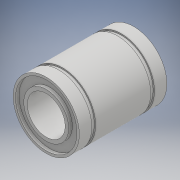
# Autodesk Inventor part: rolamento_linear_lm16uu.iam
Saved by Autodesk Inventor 2018 (Build 220112000, 112)
## iProperties
Created: 2018-05-16
Part Number: rolamento_linear_lm16uu.iam
Material: Genérico
Document SubType Name: Modeling
Designer: Usuario
Density: 1 g/cm^3
Appearance: Padrão
Mass: 6.471 g
Surface Area: 72.2059 cm^2
Volume: 6.471 cm^3
Author: Usuario
Autodesk Inventor part; units mm, degrees
ref_plane "YZ Plane" through (0, 0, 0) normal (1, 0, 0) x (0, 1, 0)
ref_plane "XZ Plane" through (0, 0, 0) normal (0, 1, 0) x (-1, 0, 0)
ref_plane "XY Plane" through (0, 0, 0) normal (0, 0, 1) x (1, 0, 0)
sketch "Esboço1" plane through (0, 0, 0) normal (0, 0, 1) x (1, 0, 0)
  line L0 (-14, 0) -> (-14, 5.25)
  line L1 (-14, 5.25) -> (-13.45, 5.25)
  line L2 (-13.45, 5.25) -> (-13.45, 6.85)
  line L3 (-13.45, 6.85) -> (-14, 6.85)
  line L4 (-14, 6.85) -> (-14, 30.15)
  line L5 (-14, 30.15) -> (-13.45, 30.15)
  line L6 (-13.45, 30.15) -> (-13.45, 31.75)
  line L7 (-13.45, 31.75) -> (-14, 31.75)
  line L8 (-14, 31.75) -> (-14, 37)
  line L9 (-14, 37) -> (-13, 37)
  line L10 (-14, 0) -> (-13, 0)
  line L11 (-13, 0) -> (0, 0) construction
  line L12 (0, 0) -> (0, 37) construction
  line L13 (0, 37) -> (-13, 37) construction
  line L14 (-13, 37) -> (-13, 0)
  dimension "d0" = 13
  dimension "d1" = 37
  dimension "d4" = 0.55
  dimension "d5" = 1.6
  dimension "d6" = 1.6
  dimension "d8" = 1
  dimension "d26" = 26.5
  dimension "d27" = 5.25
  constraints: 30 end point, 9 perpendicular, 6 point on line, 2 horizontal
  measures "d0" distance of L12.end L9.end
  measures "d1" distance of L0.start L8.end
  measures "d4" distance between parallel lines of L6 L4
  measures "d5" distance of L5.end L6.end
  measures "d6" distance of L1.end L2.end
  measures "d8" distance of L8.end L9.end
  measures "d26" distance between parallel lines of L1 L7
  measures "d27" distance of L0.start L0.end
sketch "Esboço3" plane through (0, 0, 0) normal (0, 0, 1) x (1, 0, 0)
  line L0 (0, 37) -> (0, 0) construction
  line L1 (0, 37) -> (0, 35.5) construction
  line L2 (0, 0) -> (0, 1.5) construction
  line L3 (-8, 0) -> (-8, 37)
  line L4 (-8, 0) -> (-9.5, 0)
  line L5 (-9.5, 37) -> (-8, 37)
  line L6 (-9.5, 1.5) -> (-13, 1.5)
  line L7 (-13, 1.5) -> (-13, 35.5)
  line L8 (-13, 35.5) -> (-9.5, 35.5)
  line L9 (-9.5, 0) -> (-9.5, 1.5)
  line L10 (-9.5, 35.5) -> (-9.5, 37)
  dimension "d28" = 37
  dimension "d30" = 8
  dimension "d31" = 34
  dimension "d32" = 37
  dimension "d33" = 1.5
  dimension "d34" = 5
  dimension "d36" = 1.5
  dimension "d37" = 1.5
  constraints: 22 end point, 5 perpendicular, 2 horizontal, 2 point on line, 1 parallel, 1 vertical
  measures "d28" distance of L0.start L0.end
  measures "d30" distance between parallel lines of L3 L0
  measures "d31" distance of L6.end L7.end
  measures "d32" distance of L3.start L3.end
  measures "d33" distance of L4.end L6.start
  measures "d34" distance between parallel lines of L7 L3
  measures "d36" distance of L3.start L4.end
  measures "d37" distance of L5.start L3.end
revolve "Revolução1" add sketch "Esboço3" angle 360 about axis through (0, 37, 0) along (0, -1, 0)
revolve "Revolução2" add sketch "Esboço1" angle 360 about axis through (0, 0, 0) along (0, 1, 0)
equation "\"d33\" = -0.5 * d31 + 0.5 * d32"
equation "\"d37\" = d36"
equation "\"d6\" = d5"
equation "\"d27\" = -0.5 * d26 + 0.5 * d1"
